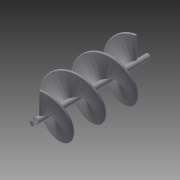
# Autodesk Inventor part: Шнек
Saved by Autodesk Inventor 2014 SP1 (Build 180222100, 222)
## iProperties
Created: 2023-07-18
Part Number: Шнек
Material: Типовые
Document SubType Name: Modeling
Designer: 1.507-7
Density: 1 g/cm^3
Appearance: По умолчанию
Author: 1.507-7
Autodesk Inventor part; units mm, degrees
ref_plane "YZ Plane" through (0, 0, 0) normal (1, 0, 0) x (0, 1, 0)
ref_plane "XZ Plane" through (0, 0, 0) normal (0, 1, 0) x (-1, 0, 0)
ref_plane "XY Plane" through (0, 0, 0) normal (0, 0, 1) x (1, 0, 0)
sketch "Эскиз1" plane through (0, 0, 0) normal (1, 0, 0) x (0, 1, 0)
  line L0 (0, 2.5) -> (0, 22.5)
  line L1 (0, 2.5) -> (2, 2.5)
  line L2 (2, 2.5) -> (2, 22.5)
  arc A0 (2, 22.5) -> (0, 22.5) centre (1, 22.5) ccw
  line L3 (-1.9367, 0) -> (5.1863, 0) construction
  point P0 (0, 0)
  dimension "d3" = 1
  constraints: 8 end point, 3 perpendicular, 2 point on circle, 2 tangent, 1 centre point, 1 vertical
  measures "d3" radius of A0
coil "Пружина1" sketch "Эскиз1" operation add axis through (0, -1.9367, 0) along (0, 1, 0) pitch 30 turns 3 hand right
sketch "Эскиз2" plane through (0, 0, 0) normal (1, 0, 0) x (0, 1, 0)
  line L0 (-3, 0) -> (97, 0)
  line L1 (97, 0) -> (97, 2.5)
  line L2 (97, 2.5) -> (-3, 2.5)
  line L3 (-3, 2.5) -> (-3, 0)
  point P0 (0, 0)
  constraints: 8 end point, 1 horizontal, 1 parallel, 1 perpendicular
revolve "Вращение1" add sketch "Эскиз2" angle 360 about axis through (0, -3, 0) along (0, 1, 0)
sketch "Эскиз4" plane through (0, -3, 0) normal (0, -1, 0) x (1, 0, 0)
  circle A0 centre (0, 0) radius 2.5 projected
  line L0 (-2.5, 0) -> (0, -2.5)
  line L1 (0, -2.5) -> (2.5, 0)
  line L2 (-2.5, 0) -> (0, 2.5)
  line L3 (0, 2.5) -> (2.5, 0)
  constraints: 8 end point, 4 point on circle, 2 perpendicular, 1 parallel
extrude "Выдавливание1" cut sketch "Эскиз4" against normal blind 8 contours L1 L0 L2 L3
sketch "Эскиз5" plane through (0, 5, 0) normal (0, -1, 0) x (1, 0, 0)
  line L0 (0, -2.5) -> (-2.5, 0) projected
  line L1 (2.5, 0) -> (0, -2.5) projected
  line L2 (0, 2.5) -> (2.5, 0) projected
  line L3 (-2.5, 0) -> (0, 2.5) projected
  point P0 (0, 0)
extrude "Выдавливание2" add sketch "Эскиз5" along normal blind 12
sketch "Эскиз6" plane through (0, 97, 0) normal (0, 1, 0) x (1, 0, 0)
  circle A0 centre (0, 0) radius 2.5 projected
extrude "Выдавливание3" add sketch "Эскиз6" along normal blind 5
